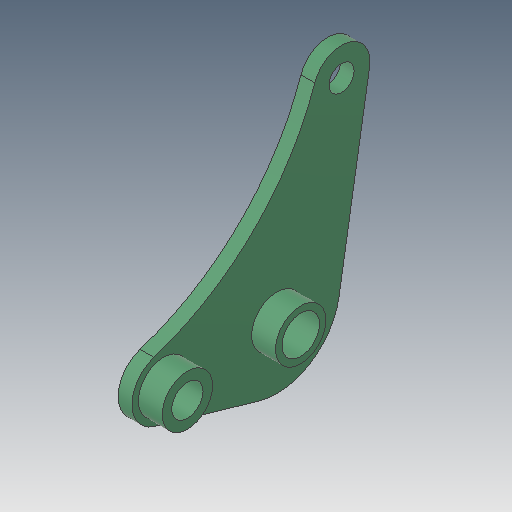
# Autodesk Inventor part: UPPER_LEG_BELT_TENSIONER
Saved by Autodesk Inventor 2019.4 (Build 234330000, 330)
## iProperties
Created: 2019-11-13
Part Number: UPPER_LEG_BELT_TENSIONER
Material: 一般
Document SubType Name: Modeling
Designer: y6tada
Density: 1 g/cm^3
Appearance: 滑らか - 濃い海緑
Mass: 0.229639 g
Surface Area: 5.47922 cm^2
Volume: 0.229639 cm^3
Author: y6tada
Autodesk Inventor part; units mm, degrees
ref_plane "YZ Plane" through (0, 0, 0) normal (1, 0, 0) x (0, 1, 0)
ref_plane "XZ Plane" through (0, 0, 0) normal (0, 1, 0) x (-1, 0, 0)
ref_plane "XY Plane" through (0, 0, 0) normal (0, 0, 1) x (1, 0, 0)
sketch "スケッチ1" plane through (0, 0, 0) normal (1, 0, 0) x (0, 1, 0)
  line L0 (0, 0) -> (0, -9) construction
  arc A0 (2.3822, 0.7584) -> (-2.4016, 0.6944) centre (0, 0) ccw
  arc A1 (-2.1018, -8.7511) -> (1.3238, -8.9021) centre (0, 0) ccw construction
  circle A2 centre (0, -9) radius 4 construction
  line L1 (-2.4016, 0.6944) -> (-4.8032, -7.6111)
  line L2 (-0.8211, -13.9321) -> (13.7727, -16.3616)
  arc A3 (0, -2.5) -> (2.3822, 0.7584) centre (0, 0) ccw construction
  arc A4 (-2.4016, 0.6944) -> (0, -2.5) centre (0, 0) ccw construction
  arc A5 (-4.8032, -7.6111) -> (-0.8211, -13.9321) centre (0, -9) ccw
  arc A6 (13.7727, -16.3616) -> (14.8724, -12.0139) centre (14.1421, -14.1421) ccw
  arc A7 (-0.8211, -13.9321) -> (-4.8032, -7.6111) centre (0, -9) ccw construction
  line L3 (0, 0) -> (14.1421, -14.1421) construction
  arc A8 (2.3822, 0.7584) -> (14.8724, -12.0139) centre (21.3237, 6.7882) ccw
  dimension "d1" = 9
  dimension "d2" = 8
  dimension "d4" = 2.5
  dimension "d39" = 5
  dimension "d48" = 2.25
  dimension "d50" = 45
  dimension "d51" = 20
  constraints: 17 point on circle, 10 tangent, 9 centre point, 8 end point, 2 coincident, 2 concentric, 2 point on line, 1 vertical
  measures "d1" distance of L0.start L0.end
  measures "d2" diameter of A2
  measures "d4" radius of A0
  measures "d39" radius of A5
  measures "d48" radius of A6
  measures "d50" angle of L0 L3
  measures "d51" distance of L0.start L3.end
extrude "押し出し1" add sketch "スケッチ1" along normal blind 1.1
sketch "スケッチ2" plane through (1.1, 0, 0) normal (1, 0, 0) x (0, 0, -1)
  circle A0 centre (0, 0) radius 2
  circle A1 centre (9, 0) radius 2
  line L0 (0, 0) -> (9, 0) construction
  arc A2 (7.6111, -4.8032) -> (13.9321, -0.8211) centre (9, 0) ccw construction
  dimension "d12" = 4
  dimension "d13" = 4
  constraints: 2 centre point, 2 end point, 1 coincident, 1 concentric, 1 horizontal
  measures "d12" diameter of A0
  measures "d13" diameter of A1
extrude "押し出し2" add sketch "スケッチ2" along normal blind 1.9
sketch "スケッチ3" plane through (1.1, 0, 0) normal (1, 0, 0) x (0, 0, -1)
  arc A0 (16.3616, 13.7727) -> (12.0139, 14.8724) centre (14.1421, 14.1421) ccw construction
  point P0 (0, 0)
  constraints: 1 coincident
hole "穴1" at (1.1, 14.1421, -14.1421) direction (-1, 0, 0) diameter 2 end through all
sketch "スケッチ4" plane through (0, 0, 0) normal (-1, 0, 0) x (0, 0, 1)
  arc A0 (0.6944, -2.4016) -> (0.7584, 2.3822) centre (0, 0) ccw construction
  arc A1 (-13.9321, -0.8211) -> (-7.6111, -4.8032) centre (-9, 0) ccw construction
  point P0 (-9, 0)
  constraints: 2 coincident
hole "穴3" at (0, 0, 0) direction (1, 0, 0) diameter 2.49 end through all
hole "穴4" at (0, 0, -9) direction (1, 0, 0) diameter 2.99 end through all
